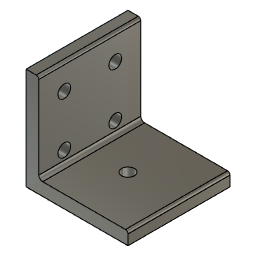
Amp Arm Fulcrum Bracket v2 (Autodesk Fusion 360 design; units mm, degrees)
Autodesk Fusion 360 part; units mm, degrees
sketch "Sketch1" plane through (0, 0, 0) normal (0, 0, 1) x (1, 0, 0)
  line L0 (-25.4, 25.4) -> (25.4, 25.4)
  line L1 (25.4, 25.4) -> (25.4, -25.4)
  line L2 (25.4, -25.4) -> (-25.4, -25.4)
  line L3 (-25.4, -25.4) -> (-25.4, 25.4)
  line L4 (0, 25.4) -> (0, -25.4)
  line L5 (-25.4, 0) -> (25.4, 0)
  circle A0 centre (0, 0) radius 3.175
  dimension "d1" = 6.35
  dimension "d2" = 50.8
  dimension "d3" = 50.8
  constraint horizontal L0
  constraint vertical L1
  constraint horizontal L2
  constraint vertical L3
  constraint midpoint L0 L4.start
  constraint midpoint L2 L4.end
  constraint midpoint L3 L5.start
  constraint midpoint L1 L5.end
  constraint coincident A0.centre origin
  measures "d1" diameter of A0
  measures "d2" distance of L4.start L4.end
  measures "d3" distance of L5.start L5.end
extrude "Extrude1" add sketch "Sketch1" along normal blind 6.35
sketch "Sketch2" plane through (0, 0, 6.35) normal (0, 0, 1) x (-1, 0, 0)
  line L0 (25.4, 25.4) -> (-25.4, 25.4)
  line L1 (-25.4, 25.4) -> (-25.4, -25.4)
  line L2 (-25.4, -25.4) -> (25.4, -25.4)
  line L3 (25.4, -25.4) -> (25.4, 25.4)
  circle A0 centre (0, 0) radius 3.175
  dimension "d6" = 6.35
  constraint coincident A0.centre origin
  measures "d6" diameter of A0
hole "Hole1" at (0, 0, 6.35) direction (0, 0, -1) diameter 6.35 depth 6.35 tip angle 118
sketch "Sketch3" plane through (0, 0, 6.35) normal (0, 0, 1) x (-1, 0, 0)
  circle A0 centre (0, 0) radius 3.175
  line L0 (25.4, 25.4) -> (-25.4, 25.4)
  line L1 (-25.4, 25.4) -> (-25.4, -25.4)
  line L2 (-25.4, -25.4) -> (25.4, -25.4)
  line L3 (25.4, -25.4) -> (25.4, 25.4)
  line L4 (19.05, -25.4) -> (19.05, 25.4)
  dimension "d10" = 6.35
  constraint coincident L2 L4.start
  constraint coincident L0 L4.end
  constraint perpendicular L0 L4
  measures "d10" distance of L3 L4.start
extrude "Extrude2" add sketch "Sketch3" along normal blind 44.45 contours L0 L2 L3 L4
sketch "Sketch4" plane through (-25.4, 0, 0) normal (-1, 0, 0) x (0, -1, 0)
  line L0 (-25.4, 0) -> (25.4, 0)
  line L1 (25.4, 0) -> (25.4, 50.8)
  line L2 (25.4, 50.8) -> (-25.4, 50.8)
  line L3 (-25.4, 50.8) -> (-25.4, 0)
  circle A0 centre (-12.7, 38.1) radius 2.3812
  circle A1 centre (12.7, 38.1) radius 2.3812
  circle A2 centre (-12.7, 12.7) radius 2.3812
  circle A3 centre (12.7, 12.7) radius 2.3812
  dimension "d13" = 4.7625
  dimension "d16" = 25.4
  dimension "d17" = -25.4
  measures "d13" diameter of A0
hole "Hole2" at (-25.4, 12.7, 38.1) at (-25.4, -12.7, 38.1) at (-25.4, -12.7, 12.7) at (-25.4, 12.7, 12.7) direction (1, 0, 0) diameter 6.35 depth 6.35 tip angle 118
sketch "Sketch5" plane through (-25.4, 0, 0) normal (-1, 0, 0) x (0, -1, 0)
  circle A0 centre (12.7, 12.7) radius 3.175
  circle A1 centre (-12.7, 38.1) radius 3.175
  circle A2 centre (12.7, 38.1) radius 3.175
  circle A3 centre (-12.7, 12.7) radius 3.175
  line L0 (-25.4, 0) -> (25.4, 0)
  line L1 (25.4, 0) -> (25.4, 50.8)
  line L2 (25.4, 50.8) -> (-25.4, 50.8)
  line L3 (-25.4, 50.8) -> (-25.4, 0)
fillet "Fillet1" radius 1.27 1 edges at (-19.05, 0, 50.8)
fillet "Fillet2" radius 1.905 1 edges at (-19.05, 0, 6.35)
fillet "Fillet3" radius 1.27 1 edges at (25.4, 0, 6.35)
equation "d13 = ( 3 / 16 ) * 1 in"
named bodies: "Amp Arm Fulcrim Bracket"
